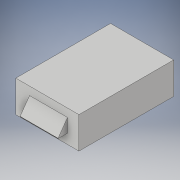
# Autodesk Inventor part: cutter grp 17-1
Saved by Autodesk Inventor 2019 (Build 230136000, 136)
## iProperties
Created: 2020-02-17
Part Number: cutter grp 17-1
Material: Generic
Document SubType Name: Modeling
Designer: Aishwarya
Density: 1 g/cm^3
Appearance: Default
Author: Aishwarya
Autodesk Inventor part; units mm, degrees
ref_plane "YZ Plane" through (0, 0, 0) normal (1, 0, 0) x (0, 1, 0)
ref_plane "XZ Plane" through (0, 0, 0) normal (0, 1, 0) x (-1, 0, 0)
ref_plane "XY Plane" through (0, 0, 0) normal (0, 0, 1) x (1, 0, 0)
sketch "Sketch1" plane through (0, 0, 0) normal (0, 0, 1) x (1, 0, 0)
  line L0 (-6.2155, 5.0202) -> (3.7845, 5.0202)
  line L1 (3.7845, 5.0202) -> (3.7845, 0.0202)
  line L2 (3.7845, 0.0202) -> (-6.2155, 0.0202)
  line L3 (-6.2155, 0.0202) -> (-6.2155, 5.0202)
  point P0 (0, 0)
  dimension "d0" = 10
  dimension "d1" = 5
  constraints: 8 end point, 2 parallel, 1 horizontal, 1 perpendicular
  measures "d0" distance of L1.end L2.end
  measures "d1" distance of L0.end L1.end
extrude "Extrusion1" add sketch "Sketch1" along normal blind 15
sketch "Sketch2" plane through (0, 0, 15) normal (0, 0, 1) x (1, 0, 0)
  line L0 (-4.0285, 3.727) -> (1.9781, 3.727)
  line L1 (1.9781, 3.727) -> (1.9781, 1.58)
  line L2 (1.9781, 1.58) -> (-4.0285, 1.58)
  line L3 (-4.0285, 1.58) -> (-4.0285, 3.727)
  point P0 (0, 0)
  constraints: 8 end point, 2 parallel, 1 horizontal, 1 perpendicular
extrude "Extrusion2" add sketch "Sketch2" along normal blind 1.5
chamfer "Chamfer1" distance 2.1 distance2 1.5 1 edges at (-1.0252, 3.727, 16.5) measured on face at (-2.0263, 3.0113, 16.5)
body "Solid1"
